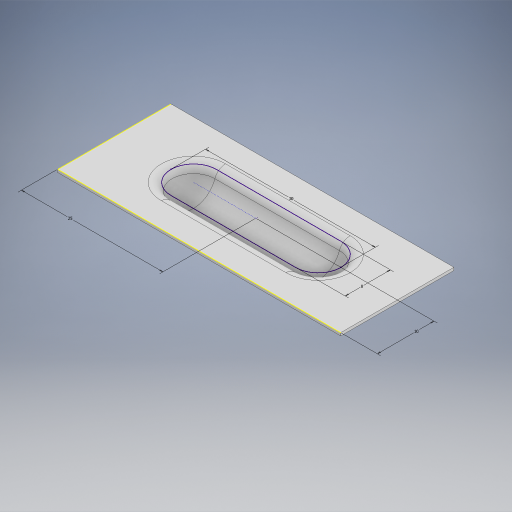
# Autodesk Inventor part: CE-4.1.4
Saved by Autodesk Inventor 2024 (Build 280153000, 153)
## iProperties
Created: 2024-02-08
Part Number: CE-4.1.4
Material: Generic
Document SubType Name: Sheet Metal
Designer: Alex
Density: 1 g/cm^3
Sheet Metal Rule: Default_mm
Appearance: Default
Author: Alex
Autodesk Inventor part; units mm, degrees
ref_plane "YZ Plane" through (0, 0, 0) normal (1, 0, 0) x (0, 1, 0)
ref_plane "XZ Plane" through (0, 0, 0) normal (0, 1, 0) x (-1, 0, 0)
sketch "Sketch1" plane through (0, 0, 0) normal (0, 1, 0) x (-1, 0, 0)
  line L0 (0, 0) -> (-50, 0)
  line L1 (-50, 0) -> (-50, -20)
  line L2 (-50, -20) -> (0, -20)
  line L3 (0, -20) -> (0, 0)
  dimension "d0" = 50
  dimension "d1" = 20
  measures "d0" distance of L2.end L1.end
  measures "d1" distance of L1.end L0.end
extrude "Plate1" add sketch "Sketch1" along normal blind 0.5
sketch "Sketch2" plane through (0, 0.5, 0) normal (0, 1, 0) x (1, 0, 0)
  line L0 (14, 10) -> (36, 10) construction
  line L1 (14, 14) -> (36, 14)
  line L2 (36, 6) -> (14, 6)
  arc A0 (14, 14) -> (14, 6) centre (14, 10) ccw
  arc A1 (36, 6) -> (36, 14) centre (36, 10) ccw
  line L3 (0, 0) -> (0, 20) projected
  line L4 (50, 0) -> (0, 0) projected
  point P0 (25, 10)
  point P1 (40, 10)
  point P2 (10, 10)
  dimension "d3" = 8
  dimension "d4" = 30
  dimension "d5" = 25
  dimension "d6" = 10
  constraints: 8 end point, 6 point on circle, 4 tangent, 2 centre point, 1 horizontal, 1 midpoint, 1 parallel
  measures "d3" distance between parallel lines of L2 L1
  measures "d4" distance of point (40, 10) point (10, 10)
  measures "d5" distance from line of L3 point (25, 10)
  measures "d6" distance from line of L4 point (25, 10)
extrude "Extrusion1" cut sketch "Sketch2" against normal blind 0.5
ref_plane "Work Plane1" through (36, 0.5, -6) normal (0, -1, 0) x (-1, 0, 0)
sketch "Sketch3" plane through (36, 0.5, -6) normal (0, -1, 0) x (-1, 0, 0)
  line L0 (0, 0) -> (22, 0) construction
  arc A0 (22, 0) -> (22, 8) centre (22, 4) ccw construction
  arc A1 (0, 8) -> (0, 0) centre (0, 4) ccw construction
  line L1 (22, 4) -> (0, 4) construction
  line L2 (26, 4) -> (-4, 4)
  arc A2 (22, 0) -> (26, 4) centre (22, 4) ccw
  arc A3 (0, 8) -> (0, 0) centre (0, 4) ccw projected
  line L3 (22, 0) -> (0, 0)
  arc A4 (-4, 4) -> (0, 0) centre (0, 4) ccw
  line L4 (26, 4) -> (26.5, 4)
  arc A5 (22, -0.5) -> (26.5, 4) centre (22, 4) ccw
  line L5 (22, -0.5) -> (0, -0.5)
  arc A6 (-4.5, 4) -> (0, -0.5) centre (0, 4) ccw
  line L6 (-4, 4) -> (-4.5, 4)
  point P0 (36, -6)
  dimension "d9" = 0.5
  constraints: 10 end point, 10 point on circle, 4 centre point, 4 horizontal, 4 tangent, 3 concentric, 1 equal radius, 1 parallel, 1 point on line, 1 vertical alignment
  measures "d9" distance of L2.start L4.end
revolve "Revolution1" add sketch "Sketch3" angle 180 about axis through (10, 0.5, -10) along (1, 0, 0) contours L4 A5 L5 A6 L6 A3 L3 A2
fillet "Fillet1" radius 2 10 edges at (38.8284, 0.5, -7.1716) (38.8284, 0.5, -12.8284) (25, 0.5, -6) (25, 0.5, -14) (11.1716, 0.5, -7.1716) (11.1716, 0.5, -12.8284) (40.4721, 0, -10) (25, 0, -5.5279) (25, 0, -14.4721) (9.5279, 0, -10)
equation "\"d7\" = Thickness"
equation "\"d9\" = Thickness"
equation "\"d2\" = Thickness"
equation "\"BendRadius\" = Thickness"
equation "\"BendReliefWidth\" = Thickness"
equation "\"BendReliefDepth\" = 0.5 * Thickness"
equation "\"CornerReliefSize\" = 4 * Thickness"
equation "\"MinimumRemnant\" = 2 * Thickness"
equation "\"TransitionRadius\" = BendRadius"
equation "\"JacobiRadiusSize\" = BendRadius"
equation "\"GapSize\" = Thickness"
equation "\"Thickness\" = 0.5"
body "Solid1"
